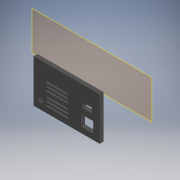
# Autodesk Inventor part: compnent box front
Saved by Autodesk Inventor 2021 (Build 250183000, 183)
## iProperties
Created: 2023-01-12
Part Number: compnent box front
Material: Generic
Document SubType Name: Modeling
Designer: boyle
Density: 1 g/cm^3
Appearance: Default
Author: boyle
Autodesk Inventor part; units mm, degrees
ref_plane "YZ Plane" through (0, 0, 0) normal (1, 0, 0) x (0, 1, 0)
ref_plane "XZ Plane" through (0, 0, 0) normal (0, 1, 0) x (-1, 0, 0)
ref_plane "XY Plane" through (0, 0, 0) normal (0, 0, 1) x (1, 0, 0)
ref_plane "Work Plane1" through (0, 0, 0) normal (0, 0, 1) x (1, 0, 0)
ref_plane "Work Plane2" through (-88.9, -98.425, 0) normal (0, 0, 1) x (1, 0, 0)
sketch "Sketch1" plane through (0, 0, 0) normal (0, 0, 1) x (1, 0, 0)
  line L0 (19.05, -98.425) -> (-88.9, -98.425) projected
  line L1 (-88.9, -98.425) -> (-88.9, -28.575) projected
  line L2 (-88.9, -28.575) -> (-88.9, 28.575) projected
  line L3 (-88.9, 28.575) -> (-85.09, 28.575) projected
  line L4 (88.9, 28.575) -> (88.9, -28.575) projected
  line L5 (85.09, 28.575) -> (88.9, 28.575) projected
  line L6 (19.05, -28.575) -> (19.05, -98.425) projected
  line L7 (-88.9, 28.575) -> (19.05, 28.575)
  line L8 (19.05, 28.575) -> (19.05, -98.425)
  line L9 (19.05, -98.425) -> (-88.9, -98.425)
  line L10 (-88.9, -98.425) -> (-88.9, 28.575)
  line L11 (15.24, -94.615) -> (-85.09, -94.615) projected
  line L12 (15.24, -94.615) -> (15.24, -28.575) projected
  line L13 (-85.09, -28.575) -> (15.24, -28.575) projected
  line L14 (-85.09, -94.615) -> (-85.09, -28.575) projected
  line L15 (19.05, -28.575) -> (19.05, -98.425) projected
  line L16 (15.24, -28.575) -> (19.05, -28.575) projected
  line L17 (-88.9, -98.425) -> (-88.9, -28.575) projected
  line L18 (19.05, -98.425) -> (-88.9, -98.425) projected
  line L19 (-88.9, 28.575) -> (88.9, 28.575) projected
  line L20 (-88.9, -28.575) -> (19.05, -28.575)
  line L21 (19.05, -28.575) -> (19.05, -98.425)
  line L22 (19.05, -98.425) -> (-88.9, -98.425)
  line L23 (-88.9, -98.425) -> (-88.9, -28.575)
  line L24 (88.9, 28.575) -> (88.9, -98.425)
  line L25 (88.9, -98.425) -> (19.05, -98.425)
  point P0 (0, 0)
  constraints: 20 end point, 4 parallel, 3 perpendicular, 2 horizontal, 1 vertical, 1 other
extrude "Extrusion1" add sketch "Sketch1" along normal blind 6.35 from surface at 0 contours L0 L1 L20 L14 L11 L12 L16 L6 | L12 L11 L14 L13
sketch "Sketch2" plane through (0, 0, 6.35) normal (0, 0, 1) x (1, 0, 0)
  line L0 (-88.9, -98.425) -> (88.9, -98.425) projected
  line L1 (-88.9, -98.425) -> (-88.9, -28.575)
  line L2 (-88.9, 28.575) -> (-88.9, -98.425) projected
  line L3 (88.9, -98.425) -> (88.9, 28.575) projected
  circle A0 centre (-77.5617, -85.1209) radius 4.0005
  line L4 (-88.9, 28.575) -> (88.9, 28.575)
  line L5 (88.9, 28.575) -> (88.9, -28.575)
  line L6 (-88.9, -28.575) -> (-88.9, 28.575)
  line L7 (88.9, 28.575) -> (-88.9, 28.575) projected
  line L8 (-9.1277, -53.833) -> (6.3663, -53.833)
  line L9 (6.3663, -53.833) -> (6.3663, -62.088)
  line L10 (6.3663, -62.088) -> (-9.1277, -62.088)
  line L11 (-9.1277, -62.088) -> (-9.1277, -53.833)
  line L12 (-9.1277, -53.833) -> (6.3663, -62.088) construction
  line L13 (6.3663, -53.833) -> (-9.1277, -62.088) construction
  line L14 (-11.2807, -71.6359) -> (8.5193, -71.6359)
  line L15 (8.5193, -71.6359) -> (8.5193, -89.4359)
  line L16 (8.5193, -89.4359) -> (-11.2807, -89.4359)
  line L17 (-11.2807, -89.4359) -> (-11.2807, -71.6359)
  line L18 (-11.2807, -71.6359) -> (8.5193, -89.4359) construction
  line L19 (8.5193, -71.6359) -> (-11.2807, -89.4359) construction
  line L20 (-68.5407, -53.088) -> (-32.5407, -53.088)
  line L21 (-32.5407, -53.088) -> (-32.5407, -89.088)
  line L22 (-32.5407, -89.088) -> (-68.5407, -89.088)
  line L23 (-68.5407, -53.088) -> (-32.5407, -89.088) construction
  line L24 (-32.5407, -53.088) -> (-68.5407, -89.088) construction
  line L25 (-68.5407, -53.088) -> (-68.5407, -89.088)
  line L26 (-50.5407, -53.088) -> (-50.5407, -56.088)
  line L27 (-50.5407, -56.088) -> (-68.5407, -56.088)
  line L28 (-50.5407, -56.088) -> (-32.5407, -56.088)
  line L29 (-50.5407, -56.088) -> (-50.5407, -59.088)
  line L30 (-50.5407, -59.088) -> (-68.5407, -59.088)
  line L31 (-50.5407, -59.088) -> (-32.5407, -59.088)
  line L32 (-50.5407, -59.088) -> (-50.5407, -62.088)
  line L33 (-50.5407, -62.088) -> (-68.5407, -62.088)
  line L34 (-50.5407, -62.088) -> (-32.5407, -62.088)
  line L35 (-50.5407, -62.088) -> (-50.5407, -65.088)
  line L36 (-50.5407, -65.088) -> (-68.5407, -65.088)
  line L37 (-50.5407, -65.088) -> (-32.5407, -65.088)
  line L38 (-50.5407, -65.088) -> (-50.5407, -68.088)
  line L39 (-50.5407, -68.088) -> (-68.5407, -68.088)
  line L40 (-50.5407, -68.088) -> (-32.5407, -68.088)
  line L41 (-50.5407, -68.088) -> (-50.5407, -71.088)
  line L42 (-50.5407, -71.088) -> (-68.5407, -71.088)
  line L43 (-50.5407, -71.088) -> (-32.5407, -71.088)
  line L44 (-50.5407, -71.088) -> (-50.5407, -74.088)
  line L45 (-50.5407, -74.088) -> (-68.5407, -74.088)
  line L46 (-50.5407, -74.088) -> (-32.5407, -74.088)
  line L47 (-50.5407, -74.088) -> (-50.5407, -77.088)
  line L48 (-50.5407, -77.088) -> (-68.5407, -77.088)
  line L49 (-50.5407, -77.088) -> (-32.5407, -77.088)
  line L50 (-50.5407, -77.088) -> (-50.5407, -80.088)
  line L51 (-50.5407, -80.088) -> (-68.5407, -80.088)
  line L52 (-50.5407, -80.088) -> (-32.5407, -80.088)
  line L53 (-50.5407, -80.088) -> (-50.5407, -83.088)
  line L54 (-50.5407, -83.088) -> (-68.5407, -83.088)
  line L55 (-50.5407, -83.088) -> (-32.5407, -83.088)
  line L56 (-50.5407, -83.088) -> (-50.5407, -86.088)
  line L57 (-50.5407, -86.088) -> (-68.5407, -86.088)
  line L58 (-50.5407, -86.088) -> (-32.5407, -86.088)
  line L59 (-50.5407, -86.088) -> (-50.5407, -89.088)
  line L60 (-50.5407, -89.088) -> (-68.5407, -89.088)
  line L61 (-50.5407, -89.088) -> (-32.5407, -89.088)
  line L62 (-11.2807, -71.6359) -> (8.5193, -71.6359)
  line L63 (8.5193, -71.6359) -> (8.5193, -89.3629)
  line L64 (8.5193, -89.3629) -> (-11.2807, -89.3629)
  line L65 (-11.2807, -89.3629) -> (-11.2807, -71.6359)
  line L66 (-9.1277, -53.833) -> (6.3663, -53.833)
  line L67 (6.3663, -53.833) -> (6.3663, -62.088)
  line L68 (6.3663, -62.088) -> (-9.1277, -62.088)
  line L69 (-9.1277, -62.088) -> (-9.1277, -53.833)
  line L70 (-68.5407, -53.088) -> (-32.5407, -53.088)
  line L71 (-32.5407, -53.088) -> (-32.5407, -89.088)
  line L72 (-32.5407, -89.088) -> (-68.5407, -89.088)
  line L73 (-68.5407, -89.088) -> (-68.5407, -53.088)
  line L74 (-68.5407, -53.088) -> (-32.5407, -53.088)
  line L75 (-32.5407, -53.088) -> (-32.5407, -56.088)
  line L76 (-32.5407, -56.088) -> (-68.5407, -56.088)
  line L77 (-68.5407, -56.088) -> (-68.5407, -53.088)
  line L78 (-68.5407, -56.088) -> (-32.5407, -56.088)
  line L79 (-32.5407, -56.088) -> (-32.5407, -59.088)
  line L80 (-32.5407, -59.088) -> (-68.5407, -59.088)
  line L81 (-68.5407, -59.088) -> (-68.5407, -56.088)
  line L82 (-32.5407, -59.088) -> (-68.5407, -59.088)
  line L83 (-68.5407, -59.088) -> (-68.5407, -62.088)
  line L84 (-68.5407, -62.088) -> (-32.5407, -62.088)
  line L85 (-32.5407, -62.088) -> (-32.5407, -59.088)
  line L86 (-68.5407, -62.088) -> (-32.5407, -62.088)
  line L87 (-32.5407, -62.088) -> (-32.5407, -65.088)
  line L88 (-32.5407, -65.088) -> (-68.5407, -65.088)
  line L89 (-68.5407, -65.088) -> (-68.5407, -62.088)
  line L90 (-32.5407, -65.088) -> (-68.5407, -65.088)
  line L91 (-68.5407, -65.088) -> (-68.5407, -68.088)
  line L92 (-68.5407, -68.088) -> (-32.5407, -68.088)
  line L93 (-32.5407, -68.088) -> (-32.5407, -65.088)
  line L94 (-68.5407, -68.088) -> (-32.5407, -68.088)
  line L95 (-32.5407, -68.088) -> (-32.5407, -71.088)
  line L96 (-32.5407, -71.088) -> (-68.5407, -71.088)
  line L97 (-68.5407, -71.088) -> (-68.5407, -68.088)
  line L98 (-32.5407, -71.088) -> (-68.5407, -71.088)
  line L99 (-68.5407, -71.088) -> (-68.5407, -74.088)
  line L100 (-68.5407, -74.088) -> (-32.5407, -74.088)
  line L101 (-32.5407, -74.088) -> (-32.5407, -71.088)
  line L102 (-68.5407, -74.088) -> (-32.5407, -74.088)
  line L103 (-32.5407, -74.088) -> (-32.5407, -77.088)
  line L104 (-32.5407, -77.088) -> (-68.5407, -77.088)
  line L105 (-68.5407, -77.088) -> (-68.5407, -74.088)
  line L106 (-32.5407, -77.088) -> (-68.5407, -77.088)
  line L107 (-68.5407, -77.088) -> (-68.5407, -79.7057)
  line L108 (-32.5407, -79.7057) -> (-32.5407, -77.088)
  line L109 (-68.5407, -77.088) -> (-32.5407, -77.088)
  line L110 (-32.5407, -77.088) -> (-32.5407, -80.088)
  line L111 (-32.5407, -80.088) -> (-68.5407, -80.088)
  line L112 (-68.5407, -80.088) -> (-68.5407, -77.088)
  line L113 (-32.5407, -80.088) -> (-68.5407, -80.088)
  line L114 (-68.5407, -80.088) -> (-68.5407, -83.088)
  line L115 (-68.5407, -83.088) -> (-32.5407, -83.088)
  line L116 (-32.5407, -83.088) -> (-32.5407, -80.088)
  line L117 (-68.5407, -83.088) -> (-32.5407, -83.088)
  line L118 (-32.5407, -83.088) -> (-32.5407, -86.088)
  line L119 (-32.5407, -86.088) -> (-68.5407, -86.088)
  line L120 (-68.5407, -86.088) -> (-68.5407, -83.088)
  line L121 (-32.5407, -86.088) -> (-68.5407, -86.088)
  line L122 (-68.5407, -86.088) -> (-68.5407, -89.088)
  line L123 (-68.5407, -89.088) -> (-32.5407, -89.088)
  line L124 (-32.5407, -89.088) -> (-32.5407, -86.088)
  line L125 (-1.3807, -80.5359) -> (-1.3807, -62.088)
  point P0 (-32.5407, -77.088)
  point P1 (-32.5407, -74.088)
  point P2 (-68.5407, -80.088)
  point P3 (-68.5407, -83.088)
  point P4 (-32.5407, -83.088)
  point P5 (-32.5407, -80.088)
  point P6 (-68.5407, -86.088)
  point P7 (-32.5407, -86.088)
  point P8 (-68.5407, -68.088)
  point P9 (-32.5407, -68.088)
  point P10 (-32.5407, -65.088)
  point P11 (-32.5407, -62.088)
  point P12 (-32.5407, -59.088)
  point P13 (-50.5407, -56.088)
  point P14 (-50.5407, -89.088)
  point P15 (-32.5407, -71.088)
  point P16 (-50.5407, -56.088)
  dimension "d2" = 69.85
  dimension "d5" = 8.001
  dimension "d8" = 15.494
  dimension "d9" = 8.255
  dimension "d12" = 19.8
  dimension "d13" = 17.8
  dimension "d34" = 36
  dimension "d35" = 36
  dimension "d39" = 3
  dimension "d40" = 3
  dimension "d41" = 3
  dimension "d42" = 3
  dimension "d43" = 3
  dimension "d44" = 3
  dimension "d45" = 3
  dimension "d46" = 3
  dimension "d47" = 3
  dimension "d48" = 3
  dimension "d49" = 3
  dimension "d50" = 3
  constraints: 244 end point, 37 parallel, 22 perpendicular, 20 horizontal, 14 vertical, 5 point on line, 2 midpoint, 1 centre point
  measures "d2" distance of L0.start L1.end
  measures "d5" diameter of A0
  measures "d8" distance of L8.start L8.end
  measures "d9" distance of L8.end L9.end
  measures "d12" distance of L14.start L14.end
  measures "d13" distance of L14.end L15.end
  measures "d34" distance of L21.end L22.end
  measures "d35" distance of L20.end L21.end
  measures "d39" distance of L26.start L26.end
  measures "d40" distance of L29.start L29.end
  measures "d41" distance of L32.start L32.end
  measures "d42" distance of L35.start L35.end
  measures "d43" distance of L38.start L38.end
  measures "d44" distance of L41.start L41.end
  measures "d45" distance of L44.start L44.end
  measures "d46" distance of L47.start L47.end
  measures "d47" distance of L50.start L50.end
  measures "d48" distance of L53.start L53.end
  measures "d49" distance of L56.start L56.end
  measures "d50" distance of L59.start L59.end
extrude "Extrusion8" cut sketch "Sketch2" against normal blind 8.001 contours A0 | L8 L9 L10 L11 | L14 L15 L64 L17 | L20 L26 L27 L25 | L20 L21 L28 L26 | L30 L32 L33 L25 | L31 L21 L34 L32 | L36 L38 L39 L25 | L37 L21 L40 L38 | L45 L47 L48 L25 | L46 L21 L49 L47 | L53 L54 L25 L51 | L52 L21 L55 L53 | L59 L22 L25 L57 | L58 L21 L22 L59
body "Solid1"
